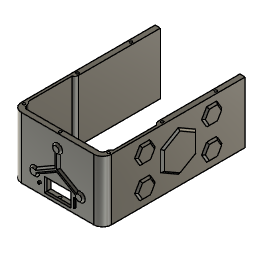
walls1 (Autodesk Fusion 360 design; units mm, degrees)
Autodesk Fusion 360 part; units mm, degrees
sketch "Sketch1" plane through (0, 0, 0) normal (0, 0, 1) x (1, 0, 0)
  line L0 (41.5, 125) -> (-41.5, 125)
  arc A0 (-41.5, 125) -> (-51.5, 115) centre (-41.5, 115) ccw
  line L1 (-51.5, 115) -> (-51.5, -130)
  arc A1 (51.5, 115) -> (41.5, 125) centre (41.5, 115) ccw
  line L2 (51.5, -130) -> (51.5, 115)
  line L3 (-41.5, -140) -> (41.5, -140)
  arc A2 (41.5, -140) -> (51.5, -130) centre (41.5, -130) ccw
  arc A3 (-51.5, -130) -> (-41.5, -140) centre (-41.5, -130) ccw
  line L4 (0, 125) -> (0, 122)
  line L5 (-51.5, 115) -> (-48.5, 115)
  circle A4 centre (-48.5, 115) radius 1.5
  circle A5 centre (0, 122) radius 1.5
  circle A6 centre (-48.5, -7.5) radius 1.5
  circle A7 centre (-48.5, 53.75) radius 1.5
  circle A8 centre (-48.5, -130) radius 1.5
  circle A9 centre (-48.5, -68.75) radius 1.5
  circle A10 centre (-48.5, -7.5) radius 1.5
  circle A11 centre (48.5, 115) radius 1.5
  circle A12 centre (48.5, 53.75) radius 1.5
  circle A13 centre (48.5, -7.5) radius 1.5
  circle A14 centre (48.5, -68.75) radius 1.5
  circle A15 centre (48.5, -130) radius 1.5
  line L6 (0, -140) -> (0, -137)
  circle A16 centre (0, -137) radius 1.5
  arc A17 (-45.5, -130) -> (-41.5, -134) centre (-41.5, -130) ccw
  line L7 (-41.5, -134) -> (41.5, -134)
  arc A18 (41.5, -134) -> (45.5, -130) centre (41.5, -130) ccw
  arc A19 (45.5, 115) -> (41.5, 119) centre (41.5, 115) ccw
  line L8 (41.5, 119) -> (-41.5, 119)
  line L9 (-48.5, -99.375) -> (-48.5, -75)
  line L10 (-48.5, -99.375) -> (-48.5, -125)
  line L11 (-45.5, 115) -> (-45.5, -75)
  line L12 (-45.5, -125) -> (-45.5, -130)
  line L13 (45.5, -130) -> (45.5, -125)
  line L14 (45.5, -75) -> (45.5, 115)
  line L15 (-48.5, -75) -> (-45.5, -75)
  line L16 (45.5, -75) -> (48.5, -75)
  line L17 (-48.5, -125) -> (-45.5, -125)
  line L18 (45.5, -125) -> (48.5, -125)
  line L19 (-48.5, -75) -> (-48.5, -125)
  line L20 (48.5, -75) -> (48.5, -125)
  arc A20 (-41.5, 119) -> (-45.5, 115) centre (-41.5, 115) ccw
  dimension "d1" = 3
  dimension "d3" = 3
  dimension "d4" = 3
  dimension "d5" = 3
  dimension "d7" = 3
  dimension "d8" = 3
  dimension "d9" = 3
  dimension "d10" = 3
  constraint midpoint L0 L4.start
  constraint perpendicular L0 L4
  constraint coincident L5.end A4.centre
  constraint coincident L4.end A5.centre
  constraint symmetric L4 A4 A11
  constraint symmetric L4 A7 A12
  constraint symmetric L4 A8 A15
  constraint symmetric L4 A9 A14
  constraint symmetric L4 A10 A13
  constraint midpoint L3 L6.start
  constraint perpendicular L3 L6
  constraint coincident L6.end A16.centre
  constraint perpendicular L10 L15
  constraint concentric A3 A17
  constraint concentric A2 A18
  constraint concentric A1 A19
  constraint tangent L7 A18
  constraint tangent A17 L7
  constraint tangent A17 L11
  constraint tangent A19 L13
  constraint tangent A18 L13
  constraint tangent A19 L8
  constraint collinear L11 L12
  constraint coincident L13.end L17
  constraint coincident L14.start L15
  constraint collinear L13 L14
  constraint collinear L15 L16
  constraint collinear L17 L18
  constraint symmetric L4 A19.start L11.start
  constraint symmetric L4 A19.end L8.end
  constraint symmetric L4 A19 A20
  measures "d1" distance of L4.start L4.end
  measures "d3" distance of A0.end L5.end
  measures "d4" diameter of A4
  measures "d5" diameter of A5
  measures "d7" diameter of A6
  measures "d8" diameter of A7
  measures "d9" distance of L6.start L6.end
  measures "d10" diameter of A16
extrude "Extrude1" add sketch "Sketch1" along normal blind 70
fillet "Fillet1" radius 5 4 edges at (45.5, -125, 35) (45.5, -75, 35) (-45.5, -75, 35) (-45.5, -125, 35)
sketch "Sketch2" plane through (0, 0, 70) normal (0, 0, 1) x (-1, 0, 0)
  arc A0 (45.5, 129.5826) -> (48.5, 125) centre (50.5, 129.5826) ccw
  line L0 (48.5, 125) -> (48.5, 75)
  arc A1 (48.5, 75) -> (45.5, 70.4174) centre (50.5, 70.4174) ccw
  line L1 (45.5, 70.4174) -> (45.5, -115)
  arc A2 (41.5, -119) -> (45.5, -115) centre (41.5, -115) ccw
  line L2 (41.5, -119) -> (-41.5, -119)
  arc A3 (-45.5, -115) -> (-41.5, -119) centre (-41.5, -115) ccw
  line L3 (-45.5, -115) -> (-45.5, 70.4174)
  arc A4 (-45.5, 70.4174) -> (-48.5, 75) centre (-50.5, 70.4174) ccw
  line L4 (-48.5, 75) -> (-48.5, 125)
  arc A5 (-48.5, 125) -> (-45.5, 129.5826) centre (-50.5, 129.5826) ccw
  line L5 (-45.5, 129.5826) -> (-45.5, 130)
  arc A6 (-41.5, 134) -> (-45.5, 130) centre (-41.5, 130) ccw
  line L6 (-41.5, 134) -> (41.5, 134)
  arc A7 (45.5, 130) -> (41.5, 134) centre (41.5, 130) ccw
  line L7 (45.5, 130) -> (45.5, 129.5826)
  circle A8 centre (48.5, -115) radius 1.5
  circle A9 centre (0, 137) radius 1.5
  circle A10 centre (0, -122) radius 1.5
  circle A11 centre (-48.5, 68.75) radius 1.5
  circle A12 centre (48.5, 130) radius 1.5
  circle A13 centre (-48.5, -115) radius 1.5
  circle A14 centre (-48.5, 130) radius 1.5
  circle A15 centre (48.5, 7.5) radius 1.5
  circle A16 centre (48.5, -53.75) radius 1.5
  circle A17 centre (-48.5, -53.75) radius 1.5
  circle A18 centre (-48.5, 7.5) radius 1.5
  circle A19 centre (48.5, 68.75) radius 1.5
  arc A20 (51.5, 130) -> (41.5, 140) centre (41.5, 130) ccw
  line L8 (41.5, 140) -> (-41.5, 140)
  arc A21 (-41.5, 140) -> (-51.5, 130) centre (-41.5, 130) ccw
  line L9 (-51.5, 130) -> (-51.5, -115)
  arc A22 (-51.5, -115) -> (-41.5, -125) centre (-41.5, -115) ccw
  line L10 (-41.5, -125) -> (41.5, -125)
  arc A23 (41.5, -125) -> (51.5, -115) centre (41.5, -115) ccw
  line L11 (51.5, -115) -> (51.5, 130)
  line L12 (48.5, -53.75) -> (48.5, 7.5)
  line L13 (-48.5, -53.75) -> (-48.5, 7.5)
  line L14 (48.5, -23.125) -> (-48.5, -23.125)
  line L15 (51.5, -23.125) -> (48.5, -23.125)
  line L16 (-48.5, -23.125) -> (-56, -23.125)
  constraint coincident A16.centre L12.start
  constraint coincident A15.centre L12.end
  constraint coincident A17.centre L13.start
  constraint coincident A18.centre L13.end
  constraint midpoint L12 L14.start
  constraint midpoint L13 L14.end
  constraint coincident L11 L15.start
  constraint perpendicular L12 L15
  constraint perpendicular L9 L16
extrude "Extrude2" cut sketch "Sketch2" against normal blind 80 contours L1 A2 L2 A3 L3 L9 A22 L10 A23 L11 L14 L15 L16
sketch "Sketch3" plane through (51.5, 0, 0) normal (1, 0, 0) x (0, 1, 0)
  line L0 (23.125, 0) -> (23.125, 70)
  line L1 (23.125, 70) -> (-130, 70)
  line L2 (-130, 70) -> (-130, 0)
  line L3 (-130, 0) -> (23.125, 0)
  line L4 (-53.4375, 70) -> (-53.4375, 0)
  line L5 (23.125, 35) -> (-130, 35)
  line L6 (-53.4375, 35) -> (-130, 70)
  line L7 (-53.4375, 35) -> (-130, 0)
  line L8 (-53.4375, 35) -> (23.125, 0)
  line L9 (-53.4375, 35) -> (23.125, 70)
  line L10 (-85.9452, 42.5) -> (-80.1717, 52.5)
  line L11 (-80.1717, 52.5) -> (-85.9452, 62.5)
  line L12 (-85.9452, 62.5) -> (-97.4923, 62.5)
  line L13 (-97.4923, 62.5) -> (-103.2658, 52.5)
  line L14 (-103.2658, 52.5) -> (-97.4923, 42.5)
  line L15 (-97.4923, 42.5) -> (-85.9452, 42.5)
  line L16 (-85.9452, 7.5) -> (-97.4923, 7.5)
  line L17 (-80.1717, 17.5) -> (-85.9452, 7.5)
  line L18 (-85.9452, 27.5) -> (-80.1717, 17.5)
  line L19 (-97.4923, 27.5) -> (-85.9452, 27.5)
  line L20 (-103.2658, 17.5) -> (-97.4923, 27.5)
  line L21 (-97.4923, 7.5) -> (-103.2658, 17.5)
  line L22 (-9.3827, 27.5) -> (-20.9298, 27.5)
  line L23 (-20.9298, 27.5) -> (-26.7033, 17.5)
  line L24 (-26.7033, 17.5) -> (-20.9298, 7.5)
  line L25 (-20.9298, 7.5) -> (-9.3827, 7.5)
  line L26 (-9.3827, 7.5) -> (-3.6092, 17.5)
  line L27 (-3.6092, 17.5) -> (-9.3827, 27.5)
  line L28 (-3.6092, 52.5) -> (-9.3827, 42.5)
  line L29 (-9.3827, 42.5) -> (-20.9298, 42.5)
  line L30 (-20.9298, 42.5) -> (-26.7033, 52.5)
  line L31 (-26.7033, 52.5) -> (-20.9298, 62.5)
  line L32 (-20.9298, 62.5) -> (-9.3827, 62.5)
  line L33 (-9.3827, 62.5) -> (-3.6092, 52.5)
  line L34 (-33.4375, 46.547) -> (-53.4375, 58.094)
  line L35 (-53.4375, 58.094) -> (-73.4375, 46.547)
  line L36 (-73.4375, 46.547) -> (-73.4375, 23.453)
  line L37 (-73.4375, 23.453) -> (-53.4375, 11.906)
  line L38 (-53.4375, 11.906) -> (-33.4375, 23.453)
  line L39 (-33.4375, 23.453) -> (-33.4375, 46.547)
  point P0 (-91.7188, 52.5)
  point P1 (-53.4375, 35)
  dimension "d18" = 10
  dimension "d19" = 20
  constraint midpoint L1 L4.start
  constraint midpoint L3 L4.end
  constraint midpoint L0 L5.start
  constraint midpoint L2 L5.end
  constraint midpoint L4 P1
  constraint coincident L1.end L2.start
  constraint coincident L2.end L3.start
  constraint coincident L0.start L3.end
  constraint coincident L0.end L1.start
  constraint midpoint L6 P0
  constraint symmetric L5 L10.start L18.start
  constraint symmetric L5 L10.end L17.start
  constraint symmetric L5 L11.end L16.start
  constraint symmetric L5 L12.end L16.end
  constraint symmetric L5 L13.end L20.start
  constraint symmetric L5 L14.end L19.start
  constraint symmetric L4 L10.start L29.end
  constraint symmetric L4 L10.end L30.end
  constraint symmetric L4 L11.end L31.end
  constraint symmetric L4 L12.end L32.end
  constraint symmetric L4 L13.end L28.start
  constraint symmetric L4 L14.end L28.end
  constraint symmetric L4 L16.start L24.end
  constraint symmetric L4 L16.end L25.end
  constraint symmetric L4 L17.start L23.end
  constraint symmetric L4 L18.start L22.end
  constraint symmetric L4 L19.start L22.start
  constraint symmetric L4 L20.start L26.end
  constraint coincident P1 L6.start
  measures "d18" distance of P0 L15
  measures "d19" distance of P1 L39
extrude "Extrude3" add sketch "Sketch3" along normal blind 2 contours L8 L23 L24 L25 L26 | L8 L22 L23 L26 L27 | L5 L8 L39 | L5 L9 L39 | L4 L7 L36 L37 | L4 L8 L38 L39 | L9 L28 L29 L30 L33 | L9 L30 L31 L32 L33 | L4 L6 L35 L36 | L5 L7 L36 | L5 L6 L36 | L4 L9 L34 L39 | L7 L18 L19 L20 L21 | L7 L16 L17 L18 L21 | L6 L10 L11 L12 L13 | L6 L10 L13 L14 L15
chamfer "Chamfer1" distance 2 angle 45 30 edges at (53.5, -63.4375, 52.3205) (53.5, -43.4375, 52.3205) (53.5, -33.4375, 35) (53.5, -43.4375, 17.6795) (53.5, -63.4375, 17.6795) (53.5, -73.4375, 35) (53.5, -91.7188, 42.5) (53.5, -83.0585, 57.5) (53.5, -100.379, 57.5) (53.5, -91.7188, 62.5) (53.5, -100.379, 47.5) (53.5, -100.379, 22.5) (53.5, -83.0585, 22.5) (53.5, -91.7188, 27.5) (53.5, -100.379, 12.5) (53.5, -91.7188, 7.5) (53.5, -83.0585, 12.5) (53.5, -83.0585, 47.5) (53.5, -15.1563, 62.5) (53.5, -6.496, 57.5) (53.5, -6.496, 47.5) (53.5, -15.1563, 42.5) (53.5, -23.8165, 47.5) (53.5, -23.8165, 57.5) (53.5, -23.8165, 22.5) (53.5, -23.8165, 12.5) (53.5, -15.1563, 7.5) (53.5, -6.496, 12.5) (53.5, -15.1563, 27.5) (53.5, -6.496, 22.5)
sketch "Sketch4" plane through (-51.5, 0, 0) normal (-1, 0, 0) x (0, -1, 0)
  line L0 (-23.125, 70) -> (-23.125, 0)
  line L1 (-23.125, 0) -> (130, 0)
  line L2 (130, 0) -> (130, 70)
  line L3 (130, 70) -> (-23.125, 70)
  line L4 (9.3827, 42.5) -> (20.9298, 42.5)
  line L5 (20.9298, 27.5) -> (26.7033, 17.5)
  line L6 (20.9298, 7.5) -> (9.3827, 7.5)
  line L7 (97.4923, 62.5) -> (103.2658, 52.5)
  line L8 (85.9452, 7.5) -> (97.4923, 7.5)
  line L9 (53.4375, 58.094) -> (33.4375, 46.547)
  line L10 (85.9452, 42.5) -> (80.1717, 52.5)
  line L11 (97.4923, 7.5) -> (103.2658, 17.5)
  line L12 (73.4375, 46.547) -> (53.4375, 58.094)
  line L13 (33.4375, 46.547) -> (33.4375, 23.453)
  line L14 (20.9298, 42.5) -> (26.7033, 52.5)
  line L15 (53.4375, 70) -> (53.4375, 0)
  line L16 (73.4375, 23.453) -> (73.4375, 46.547)
  line L17 (-23.125, 0) -> (130, 0)
  line L18 (53.4375, 35) -> (-23.125, 70)
  line L19 (53.4375, 11.906) -> (73.4375, 23.453)
  line L20 (9.3827, 7.5) -> (3.6092, 17.5)
  line L21 (103.2658, 17.5) -> (97.4923, 27.5)
  line L22 (85.9452, 62.5) -> (97.4923, 62.5)
  line L23 (85.9452, 27.5) -> (80.1717, 17.5)
  line L24 (-23.125, 70) -> (-23.125, 0)
  line L25 (103.2658, 52.5) -> (97.4923, 42.5)
  line L26 (9.3827, 27.5) -> (20.9298, 27.5)
  line L27 (3.6092, 52.5) -> (9.3827, 42.5)
  line L28 (80.1717, 52.5) -> (85.9452, 62.5)
  line L29 (53.4375, 35) -> (-23.125, 0)
  line L30 (97.4923, 27.5) -> (85.9452, 27.5)
  line L31 (80.1717, 17.5) -> (85.9452, 7.5)
  line L32 (53.4375, 35) -> (130, 70)
  line L33 (26.7033, 52.5) -> (20.9298, 62.5)
  line L34 (33.4375, 23.453) -> (53.4375, 11.906)
  line L35 (20.9298, 62.5) -> (9.3827, 62.5)
  line L36 (9.3827, 62.5) -> (3.6092, 52.5)
  line L37 (53.4375, 35) -> (130, 0)
  line L38 (130, 35) -> (-23.125, 35)
  line L39 (130, 0) -> (130, 70)
  line L40 (26.7033, 17.5) -> (20.9298, 7.5)
  line L41 (3.6092, 17.5) -> (9.3827, 27.5)
  line L42 (97.4923, 42.5) -> (85.9452, 42.5)
  line L43 (130, 70) -> (-23.125, 70)
  point P0 (15.1562, 52.5)
  point P1 (106.875, 0)
  point P2 (53.4375, 35)
  dimension "d23" = 10
  dimension "d24" = 20
  constraint midpoint L15.start L43
  constraint midpoint L15.end L17
  constraint midpoint L38.start L39
  constraint midpoint L38.end L24
  constraint midpoint P2 L15
  constraint coincident L0.start L3.end
  constraint coincident L0.end L1.start
  constraint coincident L1.end L2.start
  constraint coincident L2.end L3.start
  constraint midpoint P0 L18
  constraint symmetric L4.end L5.start L38
  constraint symmetric L14.end L5.end L38
  constraint symmetric L33.end L6.start L38
  constraint symmetric L35.end L6.end L38
  constraint symmetric L27.start L20.end L38
  constraint symmetric L4.start L26.start L38
  constraint symmetric L10.start L4.end L15
  constraint symmetric L10.end L14.end L15
  constraint symmetric L22.start L33.end L15
  constraint symmetric L7.start L35.end L15
  constraint symmetric L7.end L27.start L15
  constraint symmetric L25.end L4.start L15
  constraint symmetric L8.start L6.start L15
  constraint symmetric L8.end L6.end L15
  constraint symmetric L23.end L5.end L15
  constraint symmetric L23.start L5.start L15
  constraint symmetric L21.end L26.start L15
  constraint symmetric L11.end L20.end L15
  constraint coincident P2 L18.start
  measures "d23" distance of P0 L4
  measures "d24" distance of P2 L16
extrude "Extrude4" add sketch "Sketch4" along normal blind 2 contours L14 L18 L33 L35 L36 | L4 L14 L18 L27 L36 | L13 L29 L38 | L13 L18 L38 | L9 L13 L15 L18 | L12 L15 L16 L32 | L5 L6 L20 L29 L40 | L5 L20 L26 L29 L41 | L13 L15 L29 L34 | L15 L16 L19 L37 | L16 L37 L38 | L16 L32 L38 | L7 L10 L22 L28 L32 | L7 L10 L25 L32 L42 | L11 L21 L23 L30 L37 | L8 L11 L23 L31 L37
chamfer "Chamfer2" distance 2 angle 45 30 edges at (-53.5, -43.4375, 52.3205) (-53.5, -63.4375, 52.3205) (-53.5, -83.0585, 57.5) (-53.5, -91.7188, 62.5) (-53.5, -100.379, 57.5) (-53.5, -100.379, 47.5) (-53.5, -91.7188, 42.5) (-53.5, -83.0585, 47.5) (-53.5, -91.7188, 27.5) (-53.5, -83.0585, 22.5) (-53.5, -100.379, 22.5) (-53.5, -100.379, 12.5) (-53.5, -91.7188, 7.5) (-53.5, -83.0585, 12.5) (-53.5, -23.8165, 12.5) (-53.5, -15.1562, 7.5) (-53.5, -6.496, 12.5) (-53.5, -6.496, 22.5) (-53.5, -15.1562, 27.5) (-53.5, -23.8165, 22.5) (-53.5, -33.4375, 35) (-53.5, -43.4375, 17.6795) (-53.5, -73.4375, 35) (-53.5, -63.4375, 17.6795) (-53.5, -15.1562, 42.5) (-53.5, -23.8165, 47.5) (-53.5, -23.8165, 57.5) (-53.5, -15.1562, 62.5) (-53.5, -6.496, 57.5) (-53.5, -6.496, 47.5)
sketch "Sketch5" plane through (0, -140, 0) normal (0, -1, 0) x (1, 0, 0)
  line L0 (-41.5, 0) -> (41.5, 0)
  line L1 (41.5, 0) -> (41.5, 70)
  line L2 (41.5, 70) -> (-41.5, 70)
  line L3 (-41.5, 70) -> (-41.5, 0)
  line L4 (0, 70) -> (0, 0)
  line L5 (0, 35) -> (-25.9808, 20)
  circle A0 centre (-25.9808, 20) radius 5.5
  line L6 (-1.5, 37.5981) -> (-27.4808, 22.5981)
  circle A1 centre (0, 55) radius 5.5
  line L7 (-3, 70) -> (-3, 0)
  line L8 (1.5, 32.4019) -> (-24.4808, 17.4019)
  line L9 (3, 70) -> (3, 0)
  line L10 (1.5, 37.5981) -> (27.4808, 22.5981)
  line L11 (0, 35) -> (25.9808, 20)
  circle A2 centre (25.9808, 20) radius 5.5
  line L12 (-1.5, 32.4019) -> (24.4808, 17.4019)
  dimension "d28" = 120
  dimension "d29" = 30
  dimension "d30" = 11
  dimension "d31" = 3
  dimension "d32" = 11
  dimension "d33" = 3
  dimension "d34" = -3
  dimension "d35" = -3
  constraint midpoint L2 L4.start
  constraint coincident L4.end origin
  constraint midpoint L4 L5.start
  constraint coincident L5.end A0.centre
  constraint coincident L4 A1.centre
  constraint symmetric L4 L5.start L11.start
  constraint symmetric L4 L5.end L11.end
  constraint symmetric L4 A0 A2
  constraint symmetric L4 L6.start L10.start
  constraint symmetric L4 L6.end L10.end
  constraint symmetric L4 L8.start L12.start
  constraint symmetric L4 L8.end L12.end
  measures "d28" angle of L4 L5
  measures "d29" distance of L5.start L5.end
  measures "d30" diameter of A0
  measures "d32" diameter of A1
extrude "Extrude5" add sketch "Sketch5" along normal blind 2 contours L5 A0 L7 L8 | L4 L5 L7 L8 | L4 L9 L11 L12 | L4 L5 A1 L7 | L5 A0 L6 L7 | A0 | A1 L7 | L4 A1 L7 | L9 L11 A2 L12 | L4 A1 L9 L11 | L4 A1 L9 | L9 L10 L11 A2 | A2 | A1 L9
chamfer "Chamfer3" distance 2 angle 45 9 edges at (-13.2443, -142, 30.8175) (-10.2443, -142, 25.6214) (-30.7439, -142, 17.25) (30.7439, -142, 17.25) (10.2443, -142, 25.6214) (13.2443, -142, 30.8175) (3, -142, 43.5611) (-3, -142, 43.5611) (0, -142, 60.5)
sketch "Sketch6" plane through (0, -140, 0) normal (0, -1, 0) x (1, 0, 0)
  line L0 (0, 31.5359) -> (-20.4886, 19.7068)
  arc A0 (-23.4886, 24.903) -> (-20.4886, 19.7068) centre (-25.9808, 20) ccw
  line L1 (-23.4886, 24.903) -> (-3, 36.7321)
  line L2 (-3, 36.7321) -> (-3, 50.3902)
  arc A1 (3, 50.3902) -> (-3, 50.3902) centre (0, 55) ccw
  line L3 (3, 50.3902) -> (3, 36.7321)
  line L4 (3, 36.7321) -> (23.4886, 24.903)
  arc A2 (20.4886, 19.7068) -> (23.4886, 24.903) centre (25.9808, 20) ccw
  line L5 (20.4886, 19.7068) -> (0, 31.5359)
  line L6 (-41.5, 0) -> (41.5, 0)
  line L7 (41.5, 0) -> (41.5, 70)
  line L8 (41.5, 70) -> (-41.5, 70)
  line L9 (-41.5, 70) -> (-41.5, 0)
  line L10 (0, 0) -> (0, 5)
  line L11 (0, 5) -> (13.7, 5)
  line L12 (0, 5) -> (-13.7, 5)
  line L13 (13.7, 5) -> (13.7, 18.2)
  line L14 (-13.7, 5) -> (-13.7, 18.2)
  line L15 (13.7, 18.2) -> (-13.7, 18.2)
  dimension "d39" = 5
  dimension "d40" = 13.7
  dimension "d41" = 13.7
  dimension "d42" = 13.2
  dimension "d43" = 13.2
  constraint coincident L10.start origin
  constraint perpendicular L6 L10
  constraint perpendicular L10 L11
  constraint perpendicular L10 L12
  constraint perpendicular L11 L13
  constraint perpendicular L12 L14
  measures "d39" distance of L10.start L10.end
  measures "d40" distance of L10.end L11.end
  measures "d41" distance of L10.end L12.end
  measures "d42" distance of L11.end L13.end
  measures "d43" distance of L12.end L14.end
extrude "Extrude6" cut sketch "Sketch6" against normal blind 50 contours L11 L12 L13 L14 L15
chamfer "Chamfer4" distance 1.5 angle 45 4 edges at (0, -140, 5) (13.7, -140, 11.6) (0, -140, 18.2) (-13.7, -140, 11.6)
sketch "Sketch7" plane through (0, -140, 0) normal (0, -1, 0) x (1, 0, 0)
  line L0 (-41.5, 0) -> (41.5, 0)
  line L1 (41.5, 0) -> (41.5, 70)
  line L2 (41.5, 70) -> (-41.5, 70)
  line L3 (-41.5, 70) -> (-41.5, 0)
  line L4 (0, 31.5359) -> (-20.4886, 19.7068)
  arc A0 (-23.4886, 24.903) -> (-20.4886, 19.7068) centre (-25.9808, 20) ccw
  line L5 (-23.4886, 24.903) -> (-3, 36.7321)
  line L6 (-3, 36.7321) -> (-3, 50.3902)
  arc A1 (3, 50.3902) -> (-3, 50.3902) centre (0, 55) ccw
  line L7 (3, 50.3902) -> (3, 36.7321)
  line L8 (3, 36.7321) -> (23.4886, 24.903)
  arc A2 (20.4886, 19.7068) -> (23.4886, 24.903) centre (25.9808, 20) ccw
  line L9 (20.4886, 19.7068) -> (0, 31.5359)
  line L10 (-15.2, 19.7) -> (15.2, 19.7)
  line L11 (15.2, 19.7) -> (15.2, 3.5)
  line L12 (15.2, 3.5) -> (-15.2, 3.5)
  line L13 (-15.2, 3.5) -> (-15.2, 19.7)
  line L14 (15.2, 3.5) -> (15.2, 19.7)
  line L15 (15.2, 11.6) -> (20.2, 11.6)
  line L16 (-15.2, 11.6) -> (-20.2, 11.6)
  line L17 (20.2, 11.6) -> (20.2, 7)
  line L18 (21, 7) -> (21, 16.2)
  arc A3 (21, 16.2) -> (19.4, 16.2) centre (20.2, 16.2) ccw
  line L19 (19.4, 16.2) -> (19.4, 7)
  arc A4 (19.4, 7) -> (21, 7) centre (20.2, 7) ccw
  line L20 (20.2, 7) -> (20.2, 16.2) construction
  circle A5 centre (-20.2, 11.6) radius 1.5
  dimension "d47" = 5
  dimension "d48" = 5
  dimension "d49" = 3
  constraint coincident L11.end L12.start
  constraint coincident L10.end L11.start
  constraint midpoint L11 L15.start
  constraint perpendicular L11 L15
  constraint midpoint L13 L16.start
  constraint perpendicular L13 L16
  constraint perpendicular L15 L17
  constraint tangent L18 A3
  constraint tangent A3 L19
  constraint parallel L18 L19
  constraint tangent L19 A4
  constraint tangent L18 A4
  constraint perpendicular L15 L20
  constraint coincident L17.end A4.centre
  constraint coincident L16.end A5.centre
  measures "d47" distance of L15.start L15.end
  measures "d48" distance of L16.start L16.end
  measures "d49" diameter of A5
extrude "Extrude7" add sketch "Sketch7" along normal blind 2 contours L18 A3 L19 A4 | A5
chamfer "Chamfer5" distance 0.75 angle 45 5 edges at (21, -142, 11.6) (20.2, -142, 17) (19.4, -142, 11.6) (20.2, -142, 6.2) (-21.5985, -142, 11.0576)
